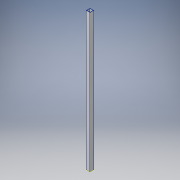
# Autodesk Inventor part: 1_250_inchSquareTube
Saved by Autodesk Inventor 2016 SP1 (Build 200210100, 210)
## iProperties
Created: 2016-01-26
Part Number: 1_250_inchSquareTube
Material: Aluminum 6061
Document SubType Name: Modeling
Designer: steele
Density: 2.7 g/cm^3
Appearance: Aluminum - Flat
Author: steele
Autodesk Inventor part; units mm, degrees
ref_plane "YZ Plane" through (0, 0, 0) normal (1, 0, 0) x (0, 1, 0)
ref_plane "XY Plane" through (0, 0, 0) normal (0, 0, 1) x (1, 0, 0)
sketch "Sketch1" plane through (0, 0, 0) normal (0, 1, 0) x (-1, 0, 0)
  line L0 (15.875, 15.875) -> (-15.875, 15.875)
  line L1 (-15.875, 15.875) -> (-15.875, -15.875)
  line L2 (-15.875, -15.875) -> (15.875, -15.875)
  line L3 (15.875, -15.875) -> (15.875, 15.875)
  line L4 (15.875, 15.875) -> (-15.875, -15.875) construction
  line L5 (-15.875, 15.875) -> (15.875, -15.875) construction
  line L6 (12.7, 12.7) -> (-12.7, 12.7)
  line L7 (-12.7, 12.7) -> (-12.7, -12.7)
  line L8 (-12.7, -12.7) -> (12.7, -12.7)
  line L9 (12.7, -12.7) -> (12.7, 12.7)
  line L10 (12.7, 12.7) -> (-12.7, -12.7) construction
  line L11 (-12.7, 12.7) -> (12.7, -12.7) construction
  point P0 (0, 0)
  dimension "d0" = 31.75
  dimension "d1" = 3.175
  constraints: 24 end point, 4 midpoint, 4 parallel, 4 perpendicular, 2 horizontal
  measures "d0" distance of L2.end L0.start
  measures "d1" distance between parallel lines of L6 L0
extrude "Extrusion1" add sketch "Sketch1" along normal blind 1143
equation "\"d0\" = tubeSize"
equation "\"d1\" = tubeThickness"
equation "\"d2\" = tubeLength"
equation "\"tubeSize\" = 31.75"
equation "\"tubeThickness\" = 3.175"
equation "\"tubeLength\" = 1143"
body "Solid1"
